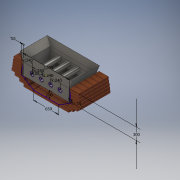
# Autodesk Inventor part: geo_pl
Saved by Autodesk Inventor 2019.1 (Build 231200000, 200)
## iProperties
Created: 2019-11-25
Part Number: geo_pl
Material: Concrete
Document SubType Name: Modeling
Designer: jjespitia
Density: 2.40731 g/cm^3
Appearance: Framing Steel
Sheet Metal Rule: Default
Author: jjespitia
Autodesk Inventor part; units mm, degrees
ref_plane "YZ Plane" through (0, 0, 0) normal (1, 0, 0) x (0, 1, 0)
ref_plane "XZ Plane" through (0, 0, 0) normal (0, 1, 0) x (-1, 0, 0)
ref_plane "XY Plane" through (0, 0, 0) normal (0, 0, 1) x (1, 0, 0)
sketch "Sketch1" plane through (0, 0, 0) normal (0, 0, 1) x (1, 0, 0)
  line L0 (-600, 0) -> (-650, -300)
  line L1 (-650, -300) -> (-325, -500)
  line L2 (-325, -500) -> (325, -500)
  line L3 (325, -500) -> (650, -300)
  line L4 (650, -300) -> (600, 0)
  line L5 (-600, 0) -> (-600, -300)
  line L6 (-600, -300) -> (600, -300)
  line L7 (600, -300) -> (600, 0)
  circle A0 centre (-360, -150) radius 54.1
  circle A1 centre (-120, -150) radius 54.1
  circle A2 centre (360, -150) radius 54.1
  circle A3 centre (120, -150) radius 54.1
  point P0 (0, 0)
  point P1 (0, -300)
  point P2 (0, -500)
  point P3 (-600, -150)
  dimension "d0" = 650
  dimension "d1" = 200
  dimension "d2" = 1200
  dimension "d3" = 50
  dimension "d4" = 50
  dimension "d5" = 300
  dimension "d75" = 108.2
  dimension "d76" = 240
  dimension "d77" = 240
  dimension "d78" = 240
  dimension "d79" = 240
  constraints: 16 end point, 7 horizontal alignment, 4 centre point, 3 equal radius, 3 midpoint, 2 perpendicular, 2 vertical alignment, 1 horizontal, 1 parallel, 1 vertical
  measures "d0" distance of L1.end L2.end
  measures "d1" distance between parallel lines of L2 L6
  measures "d2" distance of L5.end L6.end
  measures "d3" distance from line of L0.end L5
  measures "d4" distance from line of L7 L3.end
  measures "d5" distance of L6.end L4.end
  measures "d75" diameter of A0
  measures "d76" distance from line of L5 A0.centre
  measures "d77" distance of A1.centre A0.centre
  measures "d78" distance of A1.centre A3.centre
  measures "d79" distance of A2.centre A3.centre
sketch "Sketch2" plane through (0, 0, 0) normal (0, 0, 1) x (1, 0, 0)
  line L0 (-600, 0) -> (-650, -300) construction
  line L1 (-600, 0) -> (-600, -300) construction
  line L2 (-650, -300) -> (-325, -500) construction
  line L3 (-325, -500) -> (325, -500) construction
  line L4 (325, -500) -> (650, -300) construction
  line L5 (600, -300) -> (600, 0) construction
  line L6 (650, -300) -> (600, 0) construction
  line L7 (-600, -300) -> (600, -300) construction
  line L8 (2756.009, 105.6783) -> (3138.5717, 105.6783)
  line L9 (3138.5717, 105.6783) -> (3138.5717, -54.5407)
  line L10 (3138.5717, -54.5407) -> (2756.009, -54.5407)
  line L11 (2756.009, -54.5407) -> (2756.009, 105.6783)
  line L12 (-840, 0) -> (-600, 0)
  line L13 (-600, 0) -> (-600, -60)
  line L14 (-600, -60) -> (-840, -60)
  line L15 (-840, -60) -> (-840, 0)
  line L16 (600, 0) -> (600, -300) construction
  line L17 (-611.6667, -70) -> (-611.6667, -130)
  line L18 (-611.6667, -130) -> (-851.6667, -130)
  line L19 (-851.6667, -70) -> (-611.6667, -70)
  line L20 (-851.6667, -130) -> (-851.6667, -70)
  line L21 (-623.3333, -140) -> (-623.3333, -200)
  line L22 (-623.3333, -200) -> (-863.3333, -200)
  line L23 (-863.3333, -140) -> (-623.3333, -140)
  line L24 (-863.3333, -200) -> (-863.3333, -140)
  line L25 (-635, -210) -> (-635, -270)
  line L26 (-635, -270) -> (-875, -270)
  line L27 (-875, -210) -> (-635, -210)
  line L28 (-875, -270) -> (-875, -210)
  line L29 (-646.6667, -280) -> (-646.6667, -340)
  line L30 (-646.6667, -340) -> (-886.6667, -340)
  line L31 (-886.6667, -280) -> (-646.6667, -280)
  line L32 (-886.6667, -340) -> (-886.6667, -280)
  line L33 (-568.75, -350) -> (-568.75, -410)
  line L34 (-568.75, -410) -> (-808.75, -410)
  line L35 (-808.75, -350) -> (-568.75, -350)
  line L36 (-808.75, -410) -> (-808.75, -350)
  line L37 (-455, -420) -> (-455, -480)
  line L38 (-455, -480) -> (-695, -480)
  line L39 (-695, -420) -> (-455, -420)
  line L40 (-695, -480) -> (-695, -420)
  line L41 (-341.25, -490) -> (-341.25, -550)
  line L42 (-341.25, -550) -> (-581.25, -550)
  line L43 (-581.25, -490) -> (-341.25, -490)
  line L44 (-581.25, -550) -> (-581.25, -490)
  line L45 (0, -300) -> (0, -100)
  line L46 (600, 0) -> (600, -60)
  line L47 (600, -60) -> (840, -60)
  line L48 (840, 0) -> (600, 0)
  line L49 (840, -60) -> (840, 0)
  line L50 (611.6667, -70) -> (611.6667, -130)
  line L51 (611.6667, -130) -> (851.6667, -130)
  line L52 (851.6667, -70) -> (611.6667, -70)
  line L53 (851.6667, -130) -> (851.6667, -70)
  line L54 (623.3333, -140) -> (623.3333, -200)
  line L55 (623.3333, -200) -> (863.3333, -200)
  line L56 (863.3333, -140) -> (623.3333, -140)
  line L57 (863.3333, -200) -> (863.3333, -140)
  line L58 (635, -210) -> (635, -270)
  line L59 (635, -270) -> (875, -270)
  line L60 (875, -210) -> (635, -210)
  line L61 (875, -270) -> (875, -210)
  line L62 (646.6667, -280) -> (646.6667, -340)
  line L63 (646.6667, -340) -> (886.6667, -340)
  line L64 (886.6667, -280) -> (646.6667, -280)
  line L65 (568.75, -410) -> (808.75, -410)
  line L66 (808.75, -410) -> (808.75, -350)
  line L67 (808.75, -350) -> (568.75, -350)
  line L68 (568.75, -350) -> (568.75, -410)
  line L69 (886.6667, -340) -> (886.6667, -280)
  line L70 (695, -420) -> (455, -420)
  line L71 (455, -420) -> (455, -480)
  line L72 (455, -480) -> (695, -480)
  line L73 (695, -480) -> (695, -420)
  line L74 (581.25, -490) -> (341.25, -490)
  line L75 (341.25, -490) -> (341.25, -550)
  line L76 (341.25, -550) -> (581.25, -550)
  line L77 (581.25, -550) -> (581.25, -490)
  line L78 (-331.25, -500) -> (331.25, -500)
  line L79 (331.25, -500) -> (331.25, -560)
  line L80 (331.25, -560) -> (-331.25, -560)
  line L81 (-331.25, -560) -> (-331.25, -500)
  point P0 (0, 0)
  dimension "d9" = 240
  dimension "d46" = 60
  dimension "d47" = 240
  dimension "d48" = 60
  dimension "d49" = 240
  dimension "d50" = 60
  dimension "d53" = 240
  dimension "d54" = 60
  dimension "d55" = 10
  dimension "d56" = 10
  dimension "d57" = 10
  dimension "d58" = 240
  dimension "d59" = 60
  dimension "d60" = 240
  dimension "d61" = 60
  dimension "d62" = 240
  dimension "d63" = 60
  dimension "d64" = 240
  dimension "d65" = 60
  dimension "d66" = 10
  dimension "d67" = 10
  dimension "d68" = 10
  dimension "d69" = 10
  dimension "d70" = 10
  dimension "d71" = 10
  constraints: 164 end point, 31 symmetric about line, 21 parallel, 10 horizontal, 10 perpendicular, 7 point on line, 1 collinear, 1 midpoint, 1 vertical
  measures "d9" distance of L0.start L12.start
  measures "d46" distance between parallel lines of L12 L14
  measures "d47" distance of L17.start L19.start
  measures "d48" distance between parallel lines of L19 L18
  measures "d49" distance of L21.start L23.start
  measures "d50" distance between parallel lines of L23 L22
  measures "d53" distance of L25.start L27.start
  measures "d54" distance between parallel lines of L27 L26
  measures "d55" distance between parallel lines of L19 L14
  measures "d56" distance between parallel lines of L18 L23
  measures "d57" distance between parallel lines of L22 L27
  measures "d58" distance of L29.start L31.start
  measures "d59" distance between parallel lines of L31 L30
  measures "d60" distance of L35.end L36.end
  measures "d61" distance between parallel lines of L35 L34
  measures "d62" distance of L39.end L39.start
  measures "d63" distance between parallel lines of L39 L38
  measures "d64" distance of L43.end L43.start
  measures "d65" distance between parallel lines of L43 L42
  measures "d66" distance between parallel lines of L35 L30
  measures "d67" distance between parallel lines of L34 L39
  measures "d68" distance between parallel lines of L38 L43
  measures "d69" distance between parallel lines of L26 L31
  measures "d70" distance between parallel lines of L41 L81
  measures "d71" distance between parallel lines of L75 L79
extrude "Extrusion1" add sketch "Sketch2" against normal blind 120 contours L12 L13 L14 L15 | L17 L18 L20 L19 | L21 L22 L24 L23 | L25 L26 L28 L27 | L29 L30 L32 L31 | L33 L34 L36 L35 | L37 L38 L40 L39 | L41 L42 L44 L43 | L48 L49 L47 L46 | L52 L53 L51 L50 | L56 L57 L55 L54 | L60 L61 L59 L58 | L64 L69 L63 L62 | L68 L67 L66 L65 | L73 L72 L71 L70 | L77 L76 L75 L74 | L78 L79 L80 L81
pattern_linear "Rectangular Pattern1" count 6 spacing 130 along (0, 0, -1) of "Extrusion1"
sketch "Sketch3" plane through (0, 0, 0) normal (0, 0, 1) x (1, 0, 0)
  line L0 (-600, 0) -> (-600, -300) projected
  line L1 (-600, -300) -> (600, -300) projected
  line L2 (600, -300) -> (600, 0) projected
  line L3 (593.65, 0) -> (593.65, -293.65)
  line L4 (-593.65, -293.65) -> (-593.65, 0)
  line L5 (-593.65, 0) -> (-674.4552, 200)
  line L6 (-595.4835, 0) -> (-676.2888, 200)
  line L7 (-595.4835, 0) -> (-600, 0)
  line L8 (600, 0) -> (595.4835, 0)
  line L9 (595.4835, 0) -> (676.2888, 200)
  line L10 (593.65, 0) -> (674.4552, 200)
  line L11 (-674.4552, 200) -> (-676.2888, 200)
  line L12 (676.2888, 200) -> (674.4552, 200)
  line L13 (-674.4552, 200) -> (674.4552, 200) construction
  line L14 (-593.65, -293.65) -> (593.65, -293.65)
  point P0 (0, 200)
  point P1 (0, -300)
  dimension "d28" = 1.7
  dimension "d29" = 1.7
  dimension "d30" = 68
  dimension "d31" = 200
  dimension "d72" = 6.35
  dimension "d73" = 6.35
  dimension "d74" = 6.35
  constraints: 24 end point, 6 horizontal, 2 midpoint, 2 parallel, 2 vertical, 1 horizontal alignment, 1 point on line, 1 vertical alignment
  measures "d28" distance between parallel lines of L5 L6
  measures "d29" distance between parallel lines of L10 L9
  measures "d30" angle of L6 L7
  measures "d31" distance between parallel lines of L7 L11
  measures "d72" distance between parallel lines of L0 L4
  measures "d73" distance between parallel lines of L2 L3
  measures "d74" distance between parallel lines of L1 L14
extrude "Extrusion2" add sketch "Sketch3" against normal blind 700 and the other way blind 100 separate body
sketch "Sketch4" plane through (0, 0, 0) normal (0, 0, 1) x (1, 0, 0)
  line L0 (-600, 0) -> (-600, -300) projected
  line L1 (-600, -300) -> (600, -300) projected
  line L2 (600, -300) -> (600, 0) projected
  line L3 (600, 0) -> (595.4835, 0) projected
  line L4 (595.4835, 0) -> (676.2888, 200) projected
  line L5 (676.2888, 200) -> (674.4552, 200) construction
  line L6 (674.4552, 200) -> (593.65, 0) construction
  line L7 (593.65, 0) -> (593.65, -293.65) construction
  line L8 (-593.65, -293.65) -> (-593.65, 0) construction
  line L9 (-593.65, 0) -> (-674.4552, 200) construction
  line L10 (-674.4552, 200) -> (-676.2888, 200) construction
  line L11 (-676.2888, 200) -> (-595.4835, 0) projected
  line L12 (-595.4835, 0) -> (-600, 0) projected
  line L13 (-676.2888, 200) -> (676.2888, 200)
  line L14 (593.65, -293.65) -> (-593.65, -293.65) projected
  constraints: 2 end point, 2 point on line, 1 horizontal
extrude "Extrusion3" add sketch "Sketch4" along normal blind 1.7 bodies 2
sketch "Sketch5" plane through (0, 0, -700) normal (0, 0, -1) x (-1, 0, 0)
  line L0 (711.25, -210) -> (471.25, -210) projected
  line L1 (600, 0) -> (600, -100) projected
  line L2 (600, -100) -> (-600, -100) projected
  line L3 (-600, -100) -> (-600, 0) projected
  line L4 (-600, 0) -> (-595.4835, 0) projected
  line L5 (-595.4835, 0) -> (-676.2888, 200) projected
  line L6 (-676.2888, 200) -> (676.2888, 200) projected
  line L7 (676.2888, 200) -> (595.4835, 0) projected
  line L8 (595.4835, 0) -> (600, 0) projected
  point P0 (0, 0)
extrude "Extrusion4" add sketch "Sketch5" along normal blind 1.7 bodies 2
sketch "Sketch6" plane through (0, 0, 1.7) normal (0, 0, 1) x (1, 0, 0)
  line L0 (-600, 0) -> (600, 0)
  line L1 (600, 0) -> (600, -300)
  line L2 (600, -300) -> (-600, -300)
  line L3 (-600, -300) -> (-600, 0)
  point P0 (0, 0)
  constraints: 8 end point, 2 coincident, 2 parallel, 1 horizontal, 1 perpendicular
extrude "Extrusion5" add sketch "Sketch6" along normal blind 4.65 bodies 2
sketch "Sketch7" plane through (0, 0, -701.7) normal (0, 0, -1) x (-1, 0, 0)
  line L0 (-600, 0) -> (600, 0) projected
  line L1 (600, 0) -> (600, -300) projected
  line L2 (600, -300) -> (-600, -300) projected
  line L3 (-600, -300) -> (-600, 0) projected
  point P0 (0, 0)
extrude "Extrusion6" add sketch "Sketch7" along normal blind 4.65 bodies 2
extrude "Extrusion7" add sketch "Sketch1" along normal mid plane 1 separate body
sketch "Sketch8" plane through (0, 0, 6.35) normal (0, 0, 1) x (1, 0, 0)
  circle A0 centre (-360, -150) radius 54.1 projected
  circle A1 centre (-120, -150) radius 54.1 projected
  circle A2 centre (120, -150) radius 54.1 projected
  circle A3 centre (360, -150) radius 54.1 projected
  circle A4 centre (-360, -150) radius 57.15
  circle A5 centre (-120, -150) radius 57.15
  circle A6 centre (120, -150) radius 57.15
  circle A7 centre (360, -150) radius 57.15
  point P0 (0, 0)
  dimension "d80" = 3.05
  dimension "d81" = 3.05
  dimension "d82" = 3.05
  dimension "d83" = 3.05
  constraints: 4 centre point
  measures "d80" radial gap between concentric circles of A0 A4
  measures "d81" radial gap between concentric circles of A1 A5
  measures "d82" radial gap between concentric circles of A2 A6
  measures "d83" radial gap between concentric circles of A3 A7
extrude "Extrusion8" add sketch "Sketch8" against normal up to surface (712.7 mm away) bodies 2
sketch "Sketch9" plane through (0, 0, 6.35) normal (0, 0, 1) x (1, 0, 0)
  circle A0 centre (-360, -150) radius 54.1 projected
  circle A1 centre (-120, -150) radius 54.1 projected
  circle A2 centre (120, -150) radius 54.1 projected
  circle A3 centre (360, -150) radius 54.1 projected
  point P0 (0, 0)
extrude "Extrusion9" cut sketch "Sketch9" along normal through all both and the other way through all bodies 2
equation "\"d4\" = d3"
equation "\"d76\" = 0.2 * d2"
equation "\"d77\" = d76"
equation "\"d78\" = d77"
equation "\"d79\" = d77"
equation "\"BendRadius\" = Thickness"
equation "\"BendReliefWidth\" = Thickness"
equation "\"BendReliefDepth\" = 0.5 * Thickness"
equation "\"CornerReliefSize\" = 4 * Thickness"
equation "\"MinimumRemnant\" = 2 * Thickness"
equation "\"TransitionRadius\" = BendRadius"
equation "\"JacobiRadiusSize\" = Thickness"
equation "\"GapSize\" = Thickness"
equation "\"Thickness\" = 0.5"
